Autodesk Inventor part; units mm, degrees
(part 2 of 2)
sketch "Sketch5" plane through (28.4, 0, -9.3) normal (0, 0, -1) x (-1, 0, 0)
  line L0 (25.9, -17.5) -> (28.4, -17.5) projected
  line L1 (25.9, -1) -> (25.9, -17.5) projected
  line L2 (28.4, -1) -> (25.9, -1) projected
  line L3 (28.4, -17.5) -> (28.4, -66.4289) projected
  line L4 (0, 0) -> (28.4, 0) projected
  line L5 (0, -6.5) -> (0, 0) projected
  line L6 (5.2, -6.5) -> (0, -6.5) projected
  line L7 (5.2, -66.4289) -> (5.2, -6.5) projected
  line L8 (28.4, 0) -> (28.4, -1) projected
  arc A0 (11.5323, -44.1456) -> (11.4024, -51.1591) centre (19.0988, -47.7937) ccw projected
  arc A1 (24.1412, -41.0755) -> (11.5323, -44.1456) centre (16.05, -35.2722) ccw projected
  arc A2 (19.15, -56.1935) -> (24.1412, -41.0755) centre (19.0988, -47.7937) ccw projected
  arc A3 (11.4024, -51.1591) -> (19.15, -56.1935) centre (13.65, -56.1789) ccw projected
  circle A4 centre (7.9931, -50.522) radius 2.25 projected
  circle A5 centre (19.3069, -61.8357) radius 2.25 projected
  circle A6 centre (8.45, -9.75) radius 3.25
  line L9 (25.9, -6.5) -> (5.2, -6.5)
  line L10 (25.9, -1) -> (25.9, -17.5) projected
  circle A7 centre (18.45, -9.75) radius 3.25
  line L11 (5.2, -66.4289) -> (5.2, -6.5) projected
  circle A8 centre (24.4, -24.0883) radius 4
  line L12 (28.4, -17.5) -> (28.4, -66.4289) projected
  circle A9 centre (24.9, -58.1839) radius 3.5
  circle A10 centre (7.6821, -45.3169) radius 2.5
  arc A11 (24.1412, -41.0755) -> (11.5323, -44.1456) centre (16.05, -35.2722) ccw projected
  line L13 (5.2, -19.5) -> (25.9, -19.5)
  circle A12 centre (10.5284, -23) radius 3.5
  circle A13 centre (7.6821, -45.3169) radius 3
  line L14 (28.4, -66.4289) -> (5.2, -66.4289) projected
  point P0 (28.4, 0)
  point P1 (27.4, -15)
  dimension "d124" = 6.5
  dimension "d125" = 6.5
  dimension "d126" = 6.5
  dimension "d127" = 10
  dimension "d128" = 8
  dimension "d129" = 7
  dimension "d130" = 5
  dimension "d133" = 19.5
  dimension "d141" = 7
  dimension "d178" = 6
  constraints: 7 centre point, 7 tangent, 4 end point, 4 point on line, 2 perpendicular, 1 coincident, 5 other
  measures "d124" diameter of A6
  measures "d125" distance between parallel lines of L4 L9
  measures "d126" diameter of A7
  measures "d127" distance of A6.centre A7.centre
  measures "d128" diameter of A8
  measures "d129" diameter of A9
  measures "d130" diameter of A10
  measures "d133" distance between parallel lines of L13 L4
  measures "d141" diameter of A12
  measures "d178" diameter of A13
hole "Hole3" at (3.5, -58.1839, -9.3) at (4, -24.0883, -9.3) at (20.7179, -45.3169, -9.3) at (19.95, -9.75, -9.3) at (9.95, -9.75, -9.3) at (17.8716, -23, -9.3) direction (0, 0, 1) diameter 2.459 depth 10 thread size "M3x0.5" class "6H" standard "ISO Metric profile"
sketch "Sketch6" plane through (0, -66.4289, 0) normal (-1, 0, 0) x (0, 0, 1)
  line L0 (0, 40.2865) -> (0, 20.6423) projected
  line L1 (2, 18.6) -> (2, 42.7371)
  line L2 (0, 40.2865) -> (3.8, 40.2865) projected
  circle A0 centre (1.9, 30.9644) radius 1.0065 projected
  line L3 (0, 20.6423) -> (3.8, 20.6423) projected
  line L4 (3.8, 40.2865) -> (3.8, 20.6423) projected
  point P0 (0, 66.4289)
  constraints: 2 end point, 1 coincident
hole "Hole4" at (0, -35.4644, 1.9) direction (1, 0, 0) diameter 2.9 end through all countersink diameter 7 countersink angle 90 clearance for "Countersunk Flat Head Screw ISO 2009/7046" size "M2.5" standard "ISO"
sketch "Sketch8" plane through (28.4, -6.5, -9.3) normal (1, 0, 0) x (0, 0, -1)
  line L0 (-5.3, 0) -> (0, 0) projected
  line L1 (0, 0) -> (0, 6.5) projected
  line L2 (-9.3, 6.5) -> (0, 6.5) projected
  line L3 (-9.3, 0.5928) -> (-9.3, 6.5) projected
  line L4 (-5.3, 0) -> (0, 6.5)
  line L5 (-5.3, 0.5928) -> (-5.3, 0) projected
  line L6 (-9.3, 0.5928) -> (-5.3, 0.5928) projected
  line L7 (0, 0) -> (-3.1835, 2.5957)
  point P0 (-9.3, 6.5)
  point P1 (-2.65, 3.25)
  constraints: 4 end point, 1 midpoint, 1 perpendicular, 1 point on line
hole "Hole6" at (28.4, -3.25, -6.65) direction (-1, 0, 0) diameter 2.459 depth 8 thread size "M3x0.5" class "6H" standard "ISO Metric profile"
sketch "Sketch9" plane through (23.2, -66.4289, -9.3) normal (1, 0, 0) x (0, 0, -1)
  line L0 (-9.3, 0) -> (-9.3, 58.1668) projected
  line L1 (-5.3, 58.1668) -> (-9.3, 58.1668) projected
  line L2 (-9.3, 0) -> (0, 0) projected
  line L3 (0, 0) -> (0, 59.9289) projected
  line L4 (-5.3, 59.9289) -> (0, 59.9289) projected
  circle A0 centre (-3.3, 52.2136) radius 2.5
  circle A1 centre (-6.55, 2.75) radius 2.75
  circle A2 centre (-3.3, 52.2136) radius 2
  line L5 (-5.3, 46.1789) -> (-5.3, 57.1789) projected
  line L6 (-5.3, 58.1668) -> (-9.3, 58.1668) projected
  line L7 (-9.3, 0) -> (-9.3, 40.2045) projected
  line L8 (-5.3, 46.3312) -> (-5.3, 40.2045) projected
  line L9 (-9.3, 46.3312) -> (-9.3, 58.1668) projected
  line L10 (-5.3, 59.9289) -> (-5.3, 58.1668) projected
  line L11 (-9.3, 46.3312) -> (-5.3, 46.3312) projected
  line L12 (-5.3, 40.2045) -> (-9.3, 40.2045) projected
  point P0 (-9.3, 66.4289)
  point P1 (-5.3, 47.6348)
  point P2 (-4, 54.0871)
  point P3 (-9.3, 36.4371)
  point P4 (-9.3, 43.9135)
  dimension "d174" = 4
  dimension "d165" = 5
  dimension "d173" = 5.5
  constraints: 2 centre point, 1 coincident, 1 tangent, 1 vertical, 3 other
  measures "d165" diameter of A0
  measures "d173" diameter of A1
hole "Hole7" at (23.2, -14.2153, -6) at (23.2, -63.6789, -2.75) direction (-1, 0, 0) diameter 2.013 depth 10 thread size "M2.5x0.45" class "6H" standard "ISO Metric profile"
fillet "Fillet1" radius 1 1 edges at (8.5125, -8.262, -2)
hole "Hole8" at (1.9, -40.729, -9.3) at (1.9, -28.7694, -9.3) direction (0, 0, 1) diameter 1.4 end through all
sketch "Sketch12" plane through (2.5, -17.5, 0) normal (-1, 0, 0) x (0, 0, 1)
  circle A0 centre (-6.1, 10) radius 1.25 projected
  point P0 (0, 17.5)
hole "Hole9" at (2.5, -7.5, -6.1) direction (1, 0, 0) diameter 2.013 depth 10 thread size "M2.5x0.45" class "6H" standard "ISO Metric profile"
sketch "Sketch13" plane through (0, 0, -3.1) normal (0, 0, -1) x (-1, 0, 0)
  circle A0 centre (-14.75, -56.1789) radius 14.25 projected
  circle A1 centre (-14.7, -14.7) radius 14 projected
  arc A2 (-4.2588, -41.0755) -> (-16.8677, -44.1456) centre (-12.35, -35.2722) ccw projected
  arc A3 (-7.1187, -43.7444) -> (-13.101, -45.201) centre (-12.35, -35.2722) ccw projected
  circle A4 centre (-18.2726, -39.8035) radius 2.5
  circle A5 centre (-18.3164, -30.7988) radius 2.5
  circle A6 centre (-7.5461, -29.5685) radius 2.5
  circle A7 centre (-6.359, -39.7127) radius 2.5
  arc A8 (-11.186, -51.9899) -> (-12.37, -51.2205) centre (-9.3012, -47.7937) ccw projected
  point P0 (0, 0)
  point P1 (-19.4835, -42.2803)
  dimension "d206" = 5
  dimension "d207" = 5
  dimension "d215" = 5
  dimension "d216" = 5
  dimension "d218" = 1.5
  constraints: 7 tangent, 4 centre point, 1 other
  measures "d206" diameter of A4
  measures "d207" diameter of A5
  measures "d215" diameter of A6
  measures "d216" diameter of A7
hole "Hole10" at (18.2726, -39.8035, -3.1) at (18.3164, -30.7988, -3.1) at (7.5461, -29.5685, -3.1) at (6.359, -39.7127, -3.1) direction (0, 0, 1) diameter 2.7 end through all counterbore diameter 5 counterbore depth 1.1 clearance for "Countersunk Flat Head Screw ISO 2009/7046" size "M2.5" standard "ISO"
sketch "Sketch14" plane through (0, 0, -3.1) normal (0, 0, -1) x (-1, 0, 0)
  arc A0 (-8.7727, -39.0614) -> (-4.3505, -41.2013) centre (-6.359, -39.7127) ccw projected
  arc A1 (-7.8196, -37.6837) -> (-16.8499, -37.7478) centre (-12.35, -35.5681) ccw projected
  arc A2 (-20.2582, -41.3225) -> (-15.8674, -39.1217) centre (-18.2726, -39.8035) ccw projected
  arc A3 (-20.2582, -41.3225) -> (-13.101, -45.201) centre (-12.35, -35.2722) ccw projected
  arc A4 (-7.1187, -43.7444) -> (-13.101, -45.201) centre (-9.3012, -47.7937) ccw projected
  arc A5 (-7.1187, -43.7444) -> (-4.3505, -41.2013) centre (-12.35, -35.2722) ccw projected
  circle A6 centre (-18.3164, -30.7988) radius 2.5 projected
  arc A7 (-20.3166, -29.2991) -> (-20.2582, -41.3225) centre (-12.35, -35.2722) ccw projected
  arc A8 (-16.8499, -37.7478) -> (-20.2582, -41.3225) centre (-18.2726, -39.8035) ccw projected
  arc A9 (-7.8196, -37.6837) -> (-16.8499, -37.7478) centre (-12.35, -35.5681) ccw projected
  circle A10 centre (-7.5461, -29.5685) radius 2.5 projected
  arc A11 (-5.9356, -27.6563) -> (-20.3166, -29.2991) centre (-12.35, -35.2722) ccw projected
  circle A12 centre (-18.3164, -30.7988) radius 2.5 projected
  arc A13 (-7.8196, -37.6837) -> (-16.8499, -37.7478) centre (-12.35, -35.5681) ccw projected
  arc A14 (-4.3505, -41.2013) -> (-7.8196, -37.6837) centre (-6.359, -39.7127) ccw projected
  arc A15 (-4.3505, -41.2013) -> (-5.9356, -27.6563) centre (-12.35, -35.2722) ccw projected
  circle A16 centre (-7.5461, -29.5685) radius 2.5 projected
  arc A17 (-7.8196, -37.6837) -> (-16.8499, -37.7478) centre (-12.35, -35.5681) ccw projected
  line L0 (-16.2086, -41.2141) -> (-15.1712, -39.6962)
  arc A18 (-20.2582, -41.3225) -> (-15.8674, -39.1217) centre (-18.2726, -39.8035) ccw projected
  line L1 (-9.8998, -28.7257) -> (-10.6644, -30.8608)
  line L2 (-6.209, -31.6809) -> (-8.1253, -32.8939)
  line L3 (-5.5162, -37.359) -> (-7.4705, -36.6592)
  line L4 (-8.4005, -41.1557) -> (-9.464, -39.6511)
  line L5 (-18.9402, -37.3942) -> (-17.1684, -36.9033)
  line L6 (-19.1523, -33.1549) -> (-17.0623, -33.8964)
  line L7 (-16.2023, -29.4645) -> (-15.0187, -31.3398)
  circle A19 centre (-7.5461, -29.5685) radius 2.5 projected
  arc A20 (-8.7727, -39.0614) -> (-4.3505, -41.2013) centre (-6.359, -39.7127) ccw projected
  arc A21 (-4.3505, -41.2013) -> (-7.8196, -37.6837) centre (-6.359, -39.7127) ccw projected
  arc A22 (-5.9356, -27.6563) -> (-20.3166, -29.2991) centre (-12.35, -35.2722) ccw projected
  circle A23 centre (-18.3164, -30.7988) radius 2.5 projected
  arc A24 (-20.3166, -29.2991) -> (-20.2582, -41.3225) centre (-12.35, -35.2722) ccw projected
  arc A25 (-16.8499, -37.7478) -> (-20.2582, -41.3225) centre (-18.2726, -39.8035) ccw projected
  arc A26 (-8.7727, -39.0614) -> (-4.3505, -41.2013) centre (-6.359, -39.7127) ccw projected
  arc A27 (-15.8674, -39.1217) -> (-8.7727, -39.0614) centre (-12.35, -35.5681) ccw projected
  arc A28 (-20.2582, -41.3225) -> (-15.8674, -39.1217) centre (-18.2726, -39.8035) ccw projected
  arc A29 (-20.2582, -41.3225) -> (-13.101, -45.201) centre (-12.35, -35.2722) ccw projected
  arc A30 (-7.1187, -43.7444) -> (-13.101, -45.201) centre (-9.3012, -47.7937) ccw projected
  arc A31 (-7.1187, -43.7444) -> (-4.3505, -41.2013) centre (-12.35, -35.2722) ccw projected
  arc A32 (-4.3505, -41.2013) -> (-7.8196, -37.6837) centre (-6.359, -39.7127) ccw projected
  arc A33 (-4.3505, -41.2013) -> (-5.9356, -27.6563) centre (-12.35, -35.2722) ccw projected
  arc A34 (-20.3166, -29.2991) -> (-20.2582, -41.3225) centre (-12.35, -35.2722) ccw projected
  arc A35 (-16.8499, -37.7478) -> (-20.2582, -41.3225) centre (-18.2726, -39.8035) ccw projected
  arc A36 (-8.7727, -39.0614) -> (-4.3505, -41.2013) centre (-6.359, -39.7127) ccw projected
  arc A37 (-15.8674, -39.1217) -> (-8.7727, -39.0614) centre (-12.35, -35.5681) ccw projected
  arc A38 (-20.2582, -41.3225) -> (-15.8674, -39.1217) centre (-18.2726, -39.8035) ccw projected
  arc A39 (-20.2582, -41.3225) -> (-13.101, -45.201) centre (-12.35, -35.2722) ccw projected
  arc A40 (-7.1187, -43.7444) -> (-13.101, -45.201) centre (-9.3012, -47.7937) ccw projected
  arc A41 (-7.1187, -43.7444) -> (-4.3505, -41.2013) centre (-12.35, -35.2722) ccw projected
  arc A42 (-4.3505, -41.2013) -> (-7.8196, -37.6837) centre (-6.359, -39.7127) ccw projected
  arc A43 (-4.3505, -41.2013) -> (-5.9356, -27.6563) centre (-12.35, -35.2722) ccw projected
  circle A44 centre (-7.5461, -29.5685) radius 2.5 projected
  arc A45 (-5.9356, -27.6563) -> (-20.3166, -29.2991) centre (-12.35, -35.2722) ccw projected
  arc A46 (-8.7727, -39.0614) -> (-4.3505, -41.2013) centre (-6.359, -39.7127) ccw projected
  arc A47 (-15.8674, -39.1217) -> (-8.7727, -39.0614) centre (-12.35, -35.5681) ccw projected
  arc A48 (-20.2582, -41.3225) -> (-15.8674, -39.1217) centre (-18.2726, -39.8035) ccw projected
  arc A49 (-20.2582, -41.3225) -> (-13.101, -45.201) centre (-12.35, -35.2722) ccw projected
  arc A50 (-7.1187, -43.7444) -> (-13.101, -45.201) centre (-9.3012, -47.7937) ccw projected
  arc A51 (-7.1187, -43.7444) -> (-4.3505, -41.2013) centre (-12.35, -35.2722) ccw projected
  arc A52 (-4.3505, -41.2013) -> (-7.8196, -37.6837) centre (-6.359, -39.7127) ccw projected
  arc A53 (-4.3505, -41.2013) -> (-5.9356, -27.6563) centre (-12.35, -35.2722) ccw projected
  circle A54 centre (-7.5461, -29.5685) radius 2.5 projected
  arc A55 (-5.9356, -27.6563) -> (-20.3166, -29.2991) centre (-12.35, -35.2722) ccw projected
  circle A56 centre (-18.3164, -30.7988) radius 2.5 projected
  arc A57 (-20.3166, -29.2991) -> (-20.2582, -41.3225) centre (-12.35, -35.2722) ccw projected
  arc A58 (-16.8499, -37.7478) -> (-20.2582, -41.3225) centre (-18.2726, -39.8035) ccw projected
  arc A59 (-15.8674, -39.1217) -> (-8.7727, -39.0614) centre (-12.35, -35.5681) ccw projected
  point P0 (0, 0)
  point P1 (-8.1501, -37.9852)
  point P2 (-16.5433, -37.9954)
  point P3 (-16.5433, -37.9954)
  point P4 (-9.1193, -31.4561)
  point P5 (-8.1501, -37.9852)
  point P6 (-9.1193, -31.4561)
  point P7 (-16.2023, -29.4645)
  point P8 (-16.8499, -37.7478)
  point P9 (-7.8196, -37.6837)
  point P10 (-16.5433, -37.9954)
  point P11 (-15.8164, -30.7988)
  point P12 (-16.3581, -32.283)
  point P13 (-16.3581, -32.283)
  point P14 (-7.8196, -37.6837)
  point P15 (-5.0461, -29.5685)
  point P16 (-9.1193, -31.4561)
  point P17 (-9.1193, -31.4561)
  point P18 (-7.8196, -37.6837)
  point P19 (-4.3505, -41.2013)
  point P20 (-8.1501, -37.9852)
  point P21 (-7.8196, -37.6837)
  point P22 (-7.8196, -37.6837)
  point P23 (-8.7727, -39.0614)
  point P24 (-8.1584, -37.9771)
  point P25 (-7.8196, -37.6837)
  point P26 (-8.7727, -39.0614)
  constraints: 17 point on circle, 16 end point, 7 line through centre, 5 tangent, 1 coincident, 1 perpendicular, 15 other
extrude "Extrusion12" cut sketch "Sketch14" against normal up to surface (1.1 mm away) contours A0 L4 A27 | L0 A2 A27 | A14 A1 L3 | A6 | L7 A1 L6 A6 | L5 A1 A8
sketch "Sketch15" plane through (0, 0, 0) normal (0, 1, 0) x (1, 0, 0)
  line L0 (28.4, 0) -> (0, 0) projected
  line L1 (28.4, 0) -> (28.4, 9.3) projected
  line L2 (28.4, 9.3) -> (0, 9.3) projected
  line L3 (0, 0) -> (0, 9.3) projected
  line L4 (2.5, 9.3) -> (17.4, 9.3)
  line L5 (3, 9.3) -> (3, 0)
  line L6 (24.1, 9.3) -> (24.1, 0)
  line L7 (24.1, 4) -> (3, 4)
  line L8 (13.55, 0) -> (13.55, 4)
  circle A0 centre (18.825, 3) radius 3
  circle A1 centre (8.275, 3) radius 3
  line L9 (28.4, 0) -> (0, 0) projected
  dimension "d224" = 3
  dimension "d225" = 4.3
  dimension "d226" = 4
  dimension "d227" = 6
  dimension "d228" = 6
  dimension "d229" = 5.275
  dimension "d230" = 5.275
  dimension "d231" = 5.275
  dimension "d232" = 5.275
  constraints: 10 end point, 8 point on line, 4 perpendicular, 2 centre point, 2 midpoint, 2 tangent, 1 horizontal
  measures "d224" distance between parallel lines of L3 L5
  measures "d225" distance between parallel lines of L1 L6
  measures "d226" distance between parallel lines of L0 L7
  measures "d227" diameter of A0
  measures "d228" diameter of A1
  measures "d229" distance from line of L8 A1.centre
  measures "d230" distance from line of A1.centre L5
  measures "d231" distance from line of A0.centre L8
  measures "d232" distance from line of L6 A0.centre
hole "Hole11" at (18.825, 0, -3) at (8.275, 0, -3) direction (0, -1, 0) diameter 2.85 depth 8.262 thread size "M3.5x0.6" class "6H" standard "ISO Metric profile"
ref_plane "Work Plane5" through (0, 1, 0) normal (0, 1, 0) x (1, 0, 0)
sketch "Sketch16" plane through (0, 1, 0) normal (0, 1, 0) x (1, 0, 0)
  circle A0 centre (18.825, 3) radius 1.425 projected
  circle A1 centre (8.275, 3) radius 1.425 projected
  point P0 (0, 0)
hole "Hole12" at (18.825, 1, -3) at (8.275, 1, -3) direction (0, -1, 0) diameter 0.1 depth 5 countersink diameter 7 countersink angle 90
fillet "Fillet2" radius 1 6 edges at (15.1712, -39.6962, -2.55) (17.1684, -36.9033, -2.55) (17.0623, -33.8964, -2.55) (15.0187, -31.3398, -2.55) (7.4705, -36.6592, -2.55) (9.464, -39.6511, -2.55)
fillet "Fillet3" radius 5 1 edges at (7.6168, -7.7416, -0.8681)
fillet "Fillet4" radius 5 1 edges at (10.0358, -5.9072, -2)
fillet "Fillet5" radius 2 1 edges at (23.2, -26.2243, -2)
fillet "Fillet6" radius 0.5 5 edges at (11.186, -51.9899, -3.9) (12.37, -51.2205, -2.35) (12.37, -51.2205, -4.65) (13.101, -45.201, -4.65) (7.1187, -43.7444, -4.65)
body "Solid1"
